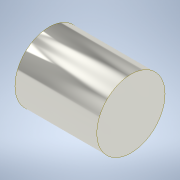
# Autodesk Inventor part: McCrea_dolny_kos_walle_MIR2
Saved by Autodesk Inventor 2022 (Build 260153000, 153)
## iProperties
Created: 2022-02-07
Part Number: McCrea_dolny_kos_walle_MIR2
Material: Generic
Document SubType Name: Modeling
Designer: student
Density: 1 g/cm^3
Appearance: Silver
Author: student
Autodesk Inventor part; units mm, degrees
ref_plane "YZ Plane" through (0, 0, 0) normal (1, 0, 0) x (0, 1, 0)
ref_plane "XZ Plane" through (0, 0, 0) normal (0, 1, 0) x (-1, 0, 0)
ref_plane "XY Plane" through (0, 0, 0) normal (0, 0, 1) x (1, 0, 0)
sketch "Sketch1" plane through (0, 0, 0) normal (0, 0, 1) x (1, 0, 0)
  line L0 (0, 0) -> (15, 0)
  line L1 (0, 0) -> (0, 7.5)
  line L2 (0, 7.5) -> (15, 7.5)
  line L3 (15, 7.5) -> (15, 0)
  dimension "d2" = 15
  constraints: 8 end point, 1 perpendicular, 1 vertical
  measures "d2" diameter of L2 L0
revolve "Revolution1" add sketch "Sketch1" angle 360 about axis through (0, 0, 0) along (1, 0, 0)
sketch "Sketch2" plane through (0, 0, 0) normal (-1, 0, 0) x (0, 0, 1)
  circle A0 centre (0, 0) radius 6.5
  circle A1 centre (0, 0) radius 7.5 projected
  dimension "d4" = 15
  dimension "d5" = 13
  constraints: 1 centre point, 1 coincident
  measures "d4" diameter of A1
  measures "d5" diameter of A0
hole "Hole1" at (0, 0, 0) direction (1, 0, 0) diameter 13 end through all
sketch "Sketch3" plane through (15, 0, 0) normal (1, 0, 0) x (0, 0, -1)
  circle A0 centre (0, 0) radius 7.5
  circle A1 centre (0, 0) radius 7.5 projected
  dimension "d13" = 15
  dimension "d14" = 15
  constraints: 1 centre point, 1 coincident
  measures "d13" diameter of A0
  measures "d14" diameter of A1
extrude "Extrusion1" add sketch "Sketch3" along normal blind 3
sketch "Sketch4" plane through (0, 0, 0) normal (-1, 0, 0) x (0, 0, 1)
  circle A0 centre (0, 0) radius 7.5 projected
  circle A1 centre (0, 0) radius 6.5 projected
  circle A2 centre (0, 0) radius 7
  line L0 (0.75, -7.25) -> (-0.75, -7.25)
  line L1 (-0.75, -7.25) -> (-0.75, -6.75)
  line L2 (-0.75, -6.75) -> (0.75, -6.75)
  line L3 (0.75, -6.75) -> (0.75, -7.25)
  line L4 (6.75, -0.75) -> (6.75, 0.75)
  line L5 (7.25, -0.75) -> (6.75, -0.75)
  line L6 (7.25, 0.75) -> (7.25, -0.75)
  line L7 (6.75, 0.75) -> (7.25, 0.75)
  line L8 (0.75, 6.75) -> (-0.75, 6.75)
  line L9 (0.75, 7.25) -> (0.75, 6.75)
  line L10 (-0.75, 7.25) -> (0.75, 7.25)
  line L11 (-0.75, 6.75) -> (-0.75, 7.25)
  line L12 (-6.75, 0.75) -> (-6.75, -0.75)
  line L13 (-7.25, 0.75) -> (-6.75, 0.75)
  line L14 (-7.25, -0.75) -> (-7.25, 0.75)
  line L15 (-6.75, -0.75) -> (-7.25, -0.75)
  dimension "d17" = 15
  dimension "d18" = 14
  dimension "d19" = 0.5
  dimension "d20" = 1.5
  dimension "d21" = 0.25
  dimension "d22" = 0.75
  dimension "d26" = 360
  constraints: 32 end point, 2 parallel, 1 centre point, 1 coincident, 1 horizontal, 1 perpendicular, 33 other
  measures "d17" diameter of A0
  measures "d18" diameter of A2
  measures "d19" distance of L2.end L0.start
  measures "d20" distance of L1.end L2.end
  measures "d21" distance edge to line of A0 L0
  measures "d22" distance from line of A0.centre L3
extrude "Extrusion2" cut sketch "Sketch4" against normal blind 3 contours A2 L5 L4 L7 | A2 L7 L6 L5 | L9 L8 L11 A2 | A2 L11 L10 L9 | L3 L0 L1 A2 | A2 L1 L2 L3 | L13 L12 L15 A2 | A2 L15 L14 L13
equation "\"d6\" = d5"
equation "\"d13\" = d14"
body "Solid1"
